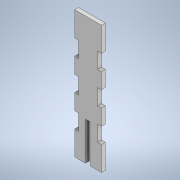
# Autodesk Inventor part: Base_1
Saved by Autodesk Inventor 2020 (Build 240168000, 168)
## iProperties
Created: 2020-12-28
Part Number: Base_1
Material: Generic
Document SubType Name: Modeling
Designer: solar
Density: 1 g/cm^3
Appearance: Default
Author: solar
Autodesk Inventor part; units mm, degrees
ref_plane "YZ Plane" through (0, 0, 0) normal (1, 0, 0) x (0, 1, 0)
ref_plane "XZ Plane" through (0, 0, 0) normal (0, 1, 0) x (-1, 0, 0)
ref_plane "XY Plane" through (0, 0, 0) normal (0, 0, 1) x (1, 0, 0)
sketch "Sketch1" plane through (0, 0, 0) normal (0, 0, 1) x (1, 0, 0)
  line L0 (-168, -100) -> (-210, -100)
  line L1 (-210, -100) -> (-210, 100)
  line L2 (-210, 100) -> (-168, 100)
  line L3 (-168, 100) -> (-168, -100)
  line L4 (-168, -100) -> (-210, 100) construction
  line L5 (-210, -100) -> (-168, 100) construction
  line L6 (-168, 0) -> (-168, 12.375)
  line L7 (-168, 12.375) -> (-174, 12.375)
  line L8 (-174, 12.375) -> (-174, -12.375)
  line L9 (-174, -12.375) -> (-168, -12.375)
  line L10 (-168, 12.375) -> (-168, 37.125)
  line L11 (-168, 37.125) -> (-174, 37.125)
  line L12 (-174, 37.125) -> (-174, 61.875)
  line L13 (-174, 61.875) -> (-168, 61.875)
  line L14 (-168, -12.375) -> (-168, -37.125)
  line L15 (-168, -37.125) -> (-174, -37.125)
  line L16 (-174, -37.125) -> (-174, -61.875)
  line L17 (-174, -61.875) -> (-168, -61.875)
  line L18 (-189, 0) -> (-189, 100)
  line L19 (-189, 0) -> (-173.1792, 0)
  line L20 (-210, 12.375) -> (-204, 12.375)
  line L21 (-204, 12.375) -> (-204, -12.375)
  line L22 (-204, -12.375) -> (-210, -12.375)
  line L23 (-210, 37.125) -> (-204, 37.125)
  line L24 (-204, 37.125) -> (-204, 61.875)
  line L25 (-204, 61.875) -> (-210, 61.875)
  line L26 (-210, -37.125) -> (-204, -37.125)
  line L27 (-204, -37.125) -> (-204, -61.875)
  line L28 (-204, -61.875) -> (-210, -61.875)
  line L29 (-185, -40) -> (-193, -40)
  line L30 (-193, -40) -> (-193, -100)
  line L31 (-193, -100) -> (-185, -100)
  line L32 (-185, -100) -> (-185, -40)
  line L33 (-185, -40) -> (-193, -100) construction
  line L34 (-193, -40) -> (-185, -100) construction
  point P0 (-210, 61.875)
  point P1 (-210, 37.125)
  point P2 (-210, 12.375)
  point P3 (-210, -12.375)
  point P4 (-210, -37.125)
  point P5 (-210, -61.875)
  point P6 (-189, -70)
  dimension "d18" = 42
  dimension "d19" = 200
  dimension "d20" = 12.375
  dimension "d21" = 6
  dimension "d22" = 24.75
  dimension "d23" = 24.75
  dimension "d24" = 6
  dimension "d25" = 24.75
  dimension "d26" = 24.75
  dimension "d27" = 6
  dimension "d28" = 24.75
  dimension "d31" = 8
  dimension "d32" = 60
  dimension "d34" = 0
  dimension "d35" = 21
  constraints: 68 end point, 12 symmetric about line, 8 perpendicular, 6 horizontal, 5 midpoint, 3 parallel, 1 vertical, 10 other
  measures "d18" distance of L1.end L2.end
  measures "d19" distance of L0.end L1.end
  measures "d20" distance of L6.start L6.end
  measures "d21" distance of L6.end L7.end
  measures "d22" distance of L7.end L8.end
  measures "d23" distance of L6.end L10.end
  measures "d24" distance of L10.end L11.end
  measures "d25" distance of L11.end L12.end
  measures "d26" distance of L9.end L14.end
  measures "d27" distance of L14.end L15.end
  measures "d28" distance of L15.end L16.end
  measures "d31" distance of L31.end L30.end
  measures "d32" distance of L30.end L29.end
  measures "d34" distance between parallel lines of L0 L31
extrude "Extrusion1" add sketch "Sketch1" along normal blind 6 contours L0 L32 L29 L30 L1 L28 L27 L26 L22 L21 L20 L23 L24 L25 L2 L18 L19 L8 L9 L3 L15 L16 L17 | L0 L30 L29 L32 | L7 L8 L19 L18 L2 L3 L13 L12 L11
extrude "Extrusion2" cut sketch "Sketch1" along normal blind 10 contours L0 L30 L29 L32
body "Solid1"
